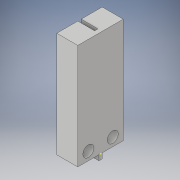
# Autodesk Inventor part: Objektträgerhalterung PHM Projekt Gegenstück
Saved by Autodesk Inventor 2017 (Build 210142000, 142)
## iProperties
Part Number: Objektträgerhalterung PHM Projekt Gegenstück
Material: Generisch
Document SubType Name: Modeling
Designer: pgmadmin
Density: 1 g/cm^3
Appearance: Vorgabe
Author: pgmadmin
Autodesk Inventor part; units mm, degrees
ref_plane "YZ Plane" through (0, 0, 0) normal (1, 0, 0) x (0, 1, 0)
ref_plane "XZ Plane" through (0, 0, 0) normal (0, 1, 0) x (-1, 0, 0)
ref_plane "XY Plane" through (0, 0, 0) normal (0, 0, 1) x (1, 0, 0)
sketch "Skizze1" plane through (0, 0, 0) normal (0, 0, 1) x (1, 0, 0)
  line L0 (-5, -10.8) -> (5, -10.8)
  line L1 (5, -10.8) -> (5, 10.8)
  line L2 (5, 10.8) -> (-5, 10.8)
  line L3 (-5, 10.8) -> (-5, -10.8)
  line L4 (-5, -10.8) -> (5, 10.8) construction
  line L5 (5, -10.8) -> (-5, 10.8) construction
  point P0 (0, 0)
  dimension "d0" = 10
  dimension "d1" = 21.6
  constraints: 12 end point, 2 midpoint, 2 parallel, 1 horizontal, 1 perpendicular
  measures "d0" distance of L1.end L2.end
  measures "d1" distance of L0.end L1.end
extrude "Extrusion1" add sketch "Skizze1" along normal blind 50
sketch "Skizze2" plane through (0, 0, 50) normal (0, 0, 1) x (1, 0, 0)
  line L0 (-5, 10.8) -> (-5, -10.8) projected
  line L1 (-5, 0.8) -> (3, 0.8)
  line L2 (3, 0.8) -> (3, -0.8)
  line L3 (3, -0.8) -> (-5, -0.8)
  line L4 (-5, -0.8) -> (-5, 0.8)
  line L5 (5, -10.8) -> (5, 10.8) projected
  point P0 (0, 0)
  dimension "d4" = 1.6
  dimension "d5" = 0.8
  dimension "d7" = 2
  constraints: 8 end point, 2 parallel, 1 horizontal, 1 perpendicular, 1 point on line
  measures "d4" distance of L1.end L2.end
  measures "d5" distance from line of point (0, 0) L1
  measures "d7" distance between parallel lines of L5 L2
extrude "Extrusion2" cut sketch "Skizze2" against normal blind 36
sketch "Skizze3" plane through (5, -10.8, 0) normal (1, 0, 0) x (0, 0, -1)
  point P0 (0, 10.8)
sketch "Skizze4" plane through (-5, 10.8, 0) normal (-1, 0, 0) x (0, 0, 1)
  line L0 (0, 0) -> (0, -21.6) projected
  line L1 (0, 0) -> (0, -21.6) projected
  line L2 (0, -21.6) -> (50, -21.6) projected
  line L3 (0, 0) -> (50, 0) projected
  circle A0 centre (4, -5) radius 2.6
  circle A1 centre (4, -16.6) radius 2.6
  point P0 (0, -10.8)
  point P1 (0, -10)
  point P2 (0, -11.6)
  dimension "d10" = 4
  dimension "d11" = 4
  dimension "d12" = 5
  dimension "d13" = 5
  dimension "d14" = 5.2
  dimension "d15" = 5.2
  constraints: 2 centre point, 2 coincident
  measures "d10" distance from line of L0 point (4, -5)
  measures "d11" distance from line of L1 point (4, -16.6)
  measures "d12" distance from line of L2 point (4, -16.6)
  measures "d13" distance from line of L3 point (4, -5)
  measures "d14" diameter of A0
  measures "d15" diameter of A1
extrude "Extrusion3" cut sketch "Skizze4" against normal blind 35
sketch "Skizze5" plane through (0, 0, 0) normal (0, 0, -1) x (-1, 0, 0)
  line L0 (-5, -0.75) -> (5, -0.75)
  line L1 (5, -0.75) -> (5, 0.75)
  line L2 (5, 0.75) -> (-5, 0.75)
  line L3 (-5, 0.75) -> (-5, -0.75)
  line L4 (-5, -10.8) -> (-5, 10.8) projected
  point P0 (0, 0)
  point P1 (-5, 0)
  dimension "d18" = 1.5
  dimension "d19" = 10
  dimension "d20" = 0
  dimension "d21" = 0.75
  constraints: 8 end point, 2 parallel, 1 horizontal, 1 midpoint, 1 perpendicular
  measures "d18" distance between parallel lines of L0 L2
  measures "d19" distance of L1.end L2.end
  measures "d20" distance between parallel lines of L3 L4
  measures "d21" distance from line of L0 point (-5, 0)
extrude "Extrusion4" add sketch "Skizze5" along normal blind 2.5
sketch "Skizze7" plane through (-5, 0.8, 50) normal (0, -1, 0) x (1, 0, 0)
  line L0 (0, -36) -> (0, 0) projected
  line L1 (10, -50) -> (0, -50)
  line L2 (0, -50) -> (0, -33.9849)
  line L3 (0, -33.9849) -> (10, -33.9849)
  line L4 (10, -33.9849) -> (10, -50)
  point P0 (5, -50)
  point P1 (0, -35)
  constraints: 8 end point, 2 parallel, 1 horizontal, 1 perpendicular, 1 point on line
extrude "Extrusion5" add sketch "Skizze7" along normal blind 2.5
sketch "Skizze8" plane through (-5, 0.8, 16.0151) normal (0, 0, 1) x (1, 0, 0)
  line L0 (0, 0) -> (8, 0) projected
  line L1 (8, -1.6) -> (0, -1.6) projected
  line L2 (8, 0) -> (0, 0)
  line L3 (0, 0) -> (0, -1.6)
  line L4 (0, -1.6) -> (8, -1.6)
  line L5 (8, -1.6) -> (8, 0)
  point P0 (5, -0.8)
  constraints: 8 end point, 2 parallel, 1 horizontal, 1 perpendicular
extrude "Extrusion6" cut sketch "Skizze8" against normal blind 1.016
